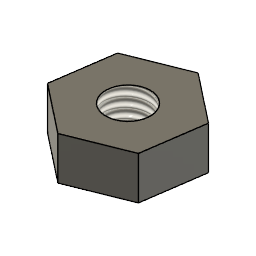
M2.5 Hexagon Nuts (Autodesk Fusion 360 design; units mm, degrees)
part number: 2026-08-01-20-47-06-922
Autodesk Fusion 360 part; units mm, degrees
sketch "Sketch1" plane through (0, 0, 0) normal (0, 1, 0) x (1, 0, 0)
  line L0 (0.4107, 2.8574) -> (-2.2692, 1.7844)
  line L1 (-2.2692, 1.7844) -> (-2.6799, -1.073)
  line L2 (-2.6799, -1.073) -> (-0.4107, -2.8574)
  line L3 (-0.4107, -2.8574) -> (2.2692, -1.7844)
  line L4 (2.2692, -1.7844) -> (2.6799, 1.073)
  line L5 (2.6799, 1.073) -> (0.4107, 2.8574)
  dimension "d1" = 2.5
  measures "d1" distance of origin L5
extrude "Extrude1" add sketch "Sketch1" along normal blind 2
sketch "Sketch2" plane through (0, 2, 0) normal (0, 1, 0) x (-1, 0, 0)
  line L0 (-2.6799, -1.073) -> (-0.4107, -2.8574)
  line L1 (-0.4107, -2.8574) -> (2.2692, -1.7844)
  line L2 (2.2692, -1.7844) -> (2.6799, 1.073)
  line L3 (2.6799, 1.073) -> (0.4107, 2.8574)
  line L4 (0.4107, 2.8574) -> (-2.2692, 1.7844)
  line L5 (-2.2692, 1.7844) -> (-2.6799, -1.073)
hole "Hole1" at (0, 2, 0) direction (0, -1, 0) diameter 2.076 depth 3.5 tip angle 118
thread "Thread1" "ISO Metric profile 2.5 M2.5x0.45 M2.5x0.45 6H" thread offset 0 thread depth 3.15
